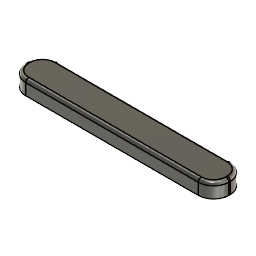
keycapX5 (Autodesk Fusion 360 design; units mm, degrees)
Autodesk Fusion 360 part; units mm, degrees
sketch "Sketch1" plane through (0, 0, 0) normal (0, 0, 1) x (1, 0, 0)
  line L0 (-0.6, 1) -> (-0.6, 2.15)
  line L1 (-0.6, 2.15) -> (0.6, 2.15)
  line L2 (0.6, 2.15) -> (0.6, 1)
  line L3 (0.9, 0.7) -> (2.15, 0.7)
  line L4 (2.15, 0.7) -> (2.15, -0.7)
  line L5 (2.15, -0.7) -> (0.9, -0.7)
  line L6 (0.6, -1) -> (0.6, -2.15)
  line L7 (0.6, -2.15) -> (-0.6, -2.15)
  line L8 (-0.6, -2.15) -> (-0.6, -1)
  line L9 (-0.9, -0.7) -> (-2.15, -0.7)
  line L10 (-2.15, -0.7) -> (-2.15, 0.7)
  line L11 (-2.15, 0.7) -> (-0.9, 0.7)
  arc A0 (-0.9, 0.7) -> (-0.6, 1) centre (-0.9, 1) ccw
  arc A1 (0.6, 1) -> (0.9, 0.7) centre (0.9, 1) ccw
  arc A2 (-0.6, -1) -> (-0.9, -0.7) centre (-0.9, -1) ccw
  arc A3 (0.9, -0.7) -> (0.6, -1) centre (0.9, -1) ccw
  circle A4 centre (0, 0) radius 3
  line L12 (28.9, 0.7) -> (30.15, 0.7)
  line L13 (27.4, 2.15) -> (28.6, 2.15)
  line L14 (28.6, -2.15) -> (27.4, -2.15)
  line L15 (30.15, 0.7) -> (30.15, -0.7)
  line L16 (25.85, -0.7) -> (25.85, 0.7)
  arc A5 (28.9, -0.7) -> (28.6, -1) centre (28.9, -1) ccw
  arc A6 (27.1, 0.7) -> (27.4, 1) centre (27.1, 1) ccw
  line L17 (28.6, 2.15) -> (28.6, 1)
  line L18 (27.4, -2.15) -> (27.4, -1)
  line L19 (30.15, -0.7) -> (28.9, -0.7)
  arc A7 (27.4, -1) -> (27.1, -0.7) centre (27.1, -1) ccw
  arc A8 (28.6, 1) -> (28.9, 0.7) centre (28.9, 1) ccw
  line L20 (27.4, 1) -> (27.4, 2.15)
  line L21 (27.1, -0.7) -> (25.85, -0.7)
  circle A9 centre (28, 0) radius 3
  line L22 (28.6, -1) -> (28.6, -2.15)
  line L23 (25.85, 0.7) -> (27.1, 0.7)
  circle A10 centre (56, 0) radius 3
  line L24 (58.15, -0.7) -> (56.9, -0.7)
  line L25 (55.4, 2.15) -> (56.6, 2.15)
  arc A11 (56.9, -0.7) -> (56.6, -1) centre (56.9, -1) ccw
  arc A12 (55.1, 0.7) -> (55.4, 1) centre (55.1, 1) ccw
  arc A13 (55.4, -1) -> (55.1, -0.7) centre (55.1, -1) ccw
  line L26 (53.85, 0.7) -> (55.1, 0.7)
  arc A14 (56.6, 1) -> (56.9, 0.7) centre (56.9, 1) ccw
  line L27 (56.9, 0.7) -> (58.15, 0.7)
  line L28 (55.4, -2.15) -> (55.4, -1)
  line L29 (56.6, 2.15) -> (56.6, 1)
  line L30 (55.1, -0.7) -> (53.85, -0.7)
  line L31 (55.4, 1) -> (55.4, 2.15)
  line L32 (58.15, 0.7) -> (58.15, -0.7)
  line L33 (53.85, -0.7) -> (53.85, 0.7)
  line L34 (56.6, -1) -> (56.6, -2.15)
  line L35 (56.6, -2.15) -> (55.4, -2.15)
  line L36 (86.15, -0.7) -> (84.9, -0.7)
  line L37 (86.15, 0.7) -> (86.15, -0.7)
  line L38 (81.85, -0.7) -> (81.85, 0.7)
  line L39 (83.4, -2.15) -> (83.4, -1)
  arc A15 (83.1, 0.7) -> (83.4, 1) centre (83.1, 1) ccw
  circle A16 centre (84, 0) radius 3
  line L40 (84.6, -1) -> (84.6, -2.15)
  line L41 (84.6, -2.15) -> (83.4, -2.15)
  line L42 (83.4, 2.15) -> (84.6, 2.15)
  line L43 (81.85, 0.7) -> (83.1, 0.7)
  arc A17 (84.6, 1) -> (84.9, 0.7) centre (84.9, 1) ccw
  line L44 (83.1, -0.7) -> (81.85, -0.7)
  arc A18 (84.9, -0.7) -> (84.6, -1) centre (84.9, -1) ccw
  arc A19 (83.4, -1) -> (83.1, -0.7) centre (83.1, -1) ccw
  line L45 (83.4, 1) -> (83.4, 2.15)
  line L46 (84.9, 0.7) -> (86.15, 0.7)
  line L47 (84.6, 2.15) -> (84.6, 1)
  line L48 (114.15, -0.7) -> (112.9, -0.7)
  line L49 (114.15, 0.7) -> (114.15, -0.7)
  line L50 (109.85, -0.7) -> (109.85, 0.7)
  line L51 (111.4, -2.15) -> (111.4, -1)
  arc A20 (111.1, 0.7) -> (111.4, 1) centre (111.1, 1) ccw
  circle A21 centre (112, 0) radius 3
  line L52 (112.6, -1) -> (112.6, -2.15)
  line L53 (112.6, -2.15) -> (111.4, -2.15)
  line L54 (111.4, 2.15) -> (112.6, 2.15)
  line L55 (109.85, 0.7) -> (111.1, 0.7)
  arc A22 (112.6, 1) -> (112.9, 0.7) centre (112.9, 1) ccw
  line L56 (111.1, -0.7) -> (109.85, -0.7)
  arc A23 (112.9, -0.7) -> (112.6, -1) centre (112.9, -1) ccw
  arc A24 (111.4, -1) -> (111.1, -0.7) centre (111.1, -1) ccw
  line L57 (111.4, 1) -> (111.4, 2.15)
  line L58 (112.9, 0.7) -> (114.15, 0.7)
  line L59 (112.6, 2.15) -> (112.6, 1)
  point P0 (0.6, 0.7)
  point P1 (28.6, 0.7)
  point P2 (28, 0)
  point P3 (56, 0)
  point P4 (56.6, 0.7)
  point P5 (84, 0)
  point P6 (84.6, 0.7)
  point P7 (112, 0)
  point P8 (112.6, 0.7)
  dimension "d2" = 4.3
  dimension "d3" = 4.3
  dimension "d4" = 2.15
  dimension "d5" = 2.15
  dimension "d6" = 1.2
  dimension "d7" = 1.4
  dimension "d8" = 0.7
  dimension "d9" = 0.6
  dimension "d10" = 0.3
  dimension "d11" = 6
  dimension "d36" = 4.3
  dimension "d37" = 4.3
  dimension "d38" = 2.15
  dimension "d39" = 2.15
  dimension "d40" = 1.2
  dimension "d41" = 1.4
  dimension "d42" = 0.7
  dimension "d43" = 0.6
  dimension "d44" = 0.3
  dimension "d45" = 6
  dimension "d46" = 28
  dimension "d47" = 4.3
  dimension "d48" = 4.3
  dimension "d49" = 2.15
  dimension "d50" = 2.15
  dimension "d51" = 1.2
  dimension "d52" = 1.4
  dimension "d53" = 0.7
  dimension "d54" = 0.6
  dimension "d55" = 0.3
  dimension "d56" = 6
  dimension "d57" = 28
  dimension "d58" = 4.3
  dimension "d59" = 4.3
  dimension "d60" = 2.15
  dimension "d61" = 2.15
  dimension "d62" = 1.2
  dimension "d63" = 1.4
  dimension "d64" = 0.7
  dimension "d65" = 0.6
  dimension "d66" = 0.3
  dimension "d67" = 6
  dimension "d68" = 4.3
  dimension "d69" = 4.3
  dimension "d70" = 2.15
  dimension "d71" = 2.15
  dimension "d72" = 1.2
  dimension "d73" = 1.4
  dimension "d74" = 0.7
  dimension "d75" = 0.6
  dimension "d76" = 0.3
  dimension "d77" = 6
  dimension "d78" = 28
  dimension "d79" = 28
  constraint vertical L0
  constraint perpendicular L0 L1
  constraint perpendicular L1 L2
  constraint perpendicular L2 L3
  constraint perpendicular L3 L4
  constraint perpendicular L4 L5
  constraint perpendicular L3 L6
  constraint perpendicular L6 L7
  constraint perpendicular L7 L8
  constraint perpendicular L8 L9
  constraint perpendicular L7 L10
  constraint perpendicular L0 L11
  constraint tangent L0 A0
  constraint tangent L11 A0
  constraint coincident P0 L2
  constraint coincident P0 L3
  constraint tangent L2 A1
  constraint tangent L3 A1
  constraint equal A0 A1
  constraint tangent L8 A2
  constraint tangent L9 A2
  constraint equal A0 A2
  constraint tangent L5 A3
  constraint tangent L6 A3
  constraint equal A0 A3
  constraint horizontal P0 L11.end
  constraint horizontal L9.start L5.end
  constraint vertical L0.start L8.end
  constraint vertical P0 L6.start
  constraint coincident A4.centre origin
  constraint vertical L20
  constraint perpendicular L13 L20
  constraint perpendicular L13 L17
  constraint perpendicular L12 L17
  constraint perpendicular L12 L15
  constraint perpendicular L15 L19
  constraint perpendicular L12 L22
  constraint perpendicular L14 L22
  constraint perpendicular L14 L18
  constraint perpendicular L18 L21
  constraint perpendicular L14 L16
  constraint perpendicular L20 L23
  constraint tangent A6 L20
  constraint tangent A6 L23
  constraint coincident P1 L17
  constraint coincident P1 L12
  constraint tangent L17 A8
  constraint tangent L12 A8
  constraint equal A6 A8
  constraint tangent L18 A7
  constraint tangent A7 L21
  constraint equal A6 A7
  constraint tangent A5 L19
  constraint tangent A5 L22
  constraint equal A5 A6
  constraint horizontal P1 A6.start
  constraint horizontal A7.end A5.start
  constraint vertical A6.end L18.end
  constraint vertical P1 A5.end
  constraint coincident P2 A9.centre
  constraint horizontal A4.centre P2
  constraint vertical L31
  constraint perpendicular L25 L31
  constraint perpendicular L25 L29
  constraint perpendicular L27 L29
  constraint perpendicular L27 L32
  constraint perpendicular L24 L32
  constraint perpendicular L27 L34
  constraint perpendicular L34 L35
  constraint perpendicular L28 L35
  constraint perpendicular L28 L30
  constraint perpendicular L33 L35
  constraint perpendicular L26 L31
  constraint tangent A12 L31
  constraint tangent A12 L26
  constraint coincident P4 L29
  constraint coincident P4 L27
  constraint tangent A14 L29
  constraint tangent A14 L27
  constraint equal A12 A14
  constraint tangent A13 L28
  constraint tangent A13 L30
  constraint equal A12 A13
  constraint tangent L24 A11
  constraint tangent A11 L34
  constraint equal A11 A12
  constraint horizontal A12.start P4
  constraint horizontal L24.end A13.end
  constraint vertical A13.start A12.end
  constraint vertical A11.end P4
  constraint coincident P3 A10.centre
  constraint horizontal P2 P3
  constraint vertical L45
  constraint perpendicular L42 L45
  constraint perpendicular L42 L47
  constraint perpendicular L46 L47
  constraint perpendicular L37 L46
  constraint perpendicular L36 L37
  constraint perpendicular L40 L46
  constraint perpendicular L40 L41
  constraint perpendicular L39 L41
  constraint perpendicular L39 L44
  constraint perpendicular L38 L41
  constraint perpendicular L43 L45
  constraint tangent A15 L45
  constraint tangent A15 L43
  constraint coincident P6 L47
  constraint coincident P6 L46
  constraint tangent A17 L47
  constraint tangent A17 L46
  constraint equal A15 A17
  constraint tangent L39 A19
  constraint tangent L44 A19
  constraint equal A15 A19
  constraint tangent L36 A18
  constraint tangent L40 A18
  constraint equal A15 A18
  constraint horizontal P6 A15.start
  constraint horizontal L44.start L36.end
  constraint vertical A15.end L39.end
  constraint vertical P6 L40.start
  constraint coincident P5 A16.centre
  constraint vertical L57
  constraint perpendicular L54 L57
  constraint perpendicular L54 L59
  constraint perpendicular L58 L59
  constraint perpendicular L49 L58
  constraint perpendicular L48 L49
  constraint perpendicular L52 L58
  constraint perpendicular L52 L53
  constraint perpendicular L51 L53
  constraint perpendicular L51 L56
  constraint perpendicular L50 L53
  constraint perpendicular L55 L57
  constraint tangent A20 L57
  constraint tangent A20 L55
  constraint coincident P8 L59
  constraint coincident P8 L58
  constraint tangent A22 L59
  constraint tangent A22 L58
  constraint equal A20 A22
  constraint tangent L51 A24
  constraint tangent L56 A24
  constraint equal A20 A24
  constraint tangent L48 A23
  constraint tangent L52 A23
  constraint equal A20 A23
  constraint horizontal P8 A20.start
  constraint horizontal L56.start L48.end
  constraint vertical A20.end L51.end
  constraint vertical P8 L52.start
  constraint coincident P7 A21.centre
  constraint horizontal P5 P7
  constraint horizontal P3 P5
  measures "d2" distance of L4 L10
  measures "d3" distance of L1 L7
  measures "d4" distance of A4.centre L4
  measures "d5" distance of A4.centre L7
  measures "d6" distance of L0.end L1.end
  measures "d7" distance of L3.end L4.end
  measures "d8" vertical distance of A4.centre P0
  measures "d9" horizontal distance of A4.centre P0
  measures "d10" radius of A0
  measures "d11" diameter of A4
  measures "d36" distance of L15 L16
  measures "d37" distance of L13 L14
  measures "d38" distance of P2 L15
  measures "d39" distance of P2 L14
  measures "d40" distance of L13.start L13.end
  measures "d41" distance of L12.end L15.end
  measures "d42" vertical distance of P1 P2
  measures "d43" horizontal distance of P1 P2
  measures "d44" radius of A6
  measures "d45" diameter of A9
  measures "d46" distance of A4.centre P2
  measures "d47" distance of L32 L33
  measures "d48" distance of L25 L35
  measures "d49" distance of P3 L32
  measures "d50" distance of P3 L35
  measures "d51" distance of L25.start L25.end
  measures "d52" distance of L27.end L24.start
  measures "d53" vertical distance of P3 P4
  measures "d54" horizontal distance of P3 P4
  measures "d55" radius of A12
  measures "d56" diameter of A10
  measures "d57" distance of P2 P3
  measures "d58" distance of L37 L38
  measures "d59" distance of L41 L42
  measures "d60" distance of P5 L37
  measures "d61" distance of P5 L41
  measures "d62" distance of L42.start L42.end
  measures "d63" distance of L36.start L37.start
  measures "d64" vertical distance of P5 P6
  measures "d65" horizontal distance of P5 P6
  measures "d66" radius of A15
  measures "d67" diameter of A16
  measures "d68" distance of L49 L50
  measures "d69" distance of L53 L54
  measures "d70" distance of P7 L49
  measures "d71" distance of P7 L53
  measures "d72" distance of L54.start L54.end
  measures "d73" distance of L48.start L49.start
  measures "d74" vertical distance of P7 P8
  measures "d75" horizontal distance of P7 P8
  measures "d76" radius of A20
  measures "d77" diameter of A21
  measures "d78" distance of P3 P5
  measures "d79" distance of P5 P7
extrude "Extrude1" add sketch "Sketch1" along normal blind 7 makes body 1 at (2.9851, -0.2987, 4.6667) makes body 2 at (30.9851, -0.2987, 4.6667) makes body 3 at (58.9851, -0.2987, 4.6667) makes body 4 at (84.9555, 2.8438, 4.6667) makes body 5 at (110.6314, -2.6696, 2.3333)
sketch "Sketch2" plane through (0, 0, 7) normal (0, 0, 1) x (-1, 0, 0)
  line L0 (-2.15, 0.7) -> (-0.9, 0.7)
  arc A0 (-0.9, 0.7) -> (-0.6, 1) centre (-0.9, 1) ccw
  line L1 (-0.6, 1) -> (-0.6, 2.15)
  line L2 (-0.6, 2.15) -> (0.6, 2.15)
  line L3 (0.6, 2.15) -> (0.6, 1)
  arc A1 (0.6, 1) -> (0.9, 0.7) centre (0.9, 1) ccw
  line L4 (0.9, 0.7) -> (2.15, 0.7)
  line L5 (2.15, 0.7) -> (2.15, -0.7)
  line L6 (2.15, -0.7) -> (0.9, -0.7)
  arc A2 (0.9, -0.7) -> (0.6, -1) centre (0.9, -1) ccw
  line L7 (0.6, -1) -> (0.6, -2.15)
  line L8 (0.6, -2.15) -> (-0.6, -2.15)
  line L9 (-0.6, -2.15) -> (-0.6, -1)
  arc A3 (-0.6, -1) -> (-0.9, -0.7) centre (-0.9, -1) ccw
  line L10 (-0.9, -0.7) -> (-2.15, -0.7)
  line L11 (-2.15, -0.7) -> (-2.15, 0.7)
  circle A4 centre (0, 0) radius 3
  line L12 (10.5, 10.5) -> (-122.5, 10.5)
  line L13 (-122.5, 10.5) -> (-122.5, -10.5)
  line L14 (-122.5, -10.5) -> (10.5, -10.5)
  line L15 (10.5, -10.5) -> (10.5, 10.5)
  dimension "d14" = 133
  dimension "d15" = 21
  dimension "d16" = 10.5
  dimension "d17" = 10.5
  constraint horizontal L12
  constraint vertical L13
  constraint horizontal L14
  constraint vertical L15
  measures "d14" distance of L12.start L12.end
  measures "d15" distance of L12.start L14.end
  measures "d16" horizontal distance of A4.centre L12.start
  measures "d17" vertical distance of A4.centre L12.start
extrude "Extrude2" add sketch "Sketch2" along normal blind 2 contours L0 A0 L1 L2 L3 A1 L4 L5 L6 A2 L7 L8 L9 A3 L10 L11 | A4 | L12 L13 L14 L15 bodies 1 2
sketch "Sketch3" plane through (0, 0, 7) normal (0, 0, -1) x (1, 0, 0)
  line L0 (-10.5, 10.5) -> (-10.5, -10.5)
  line L1 (-10.5, -10.5) -> (122.5, -10.5)
  line L2 (122.5, -10.5) -> (122.5, 10.5)
  line L3 (122.5, 10.5) -> (-10.5, 10.5)
  circle A0 centre (0, 0) radius 3
  line L4 (122.5, -10.5) -> (-10.5, -10.5)
  line L5 (-10.5, -10.5) -> (-10.5, 10.5)
  line L6 (-10.5, 10.5) -> (122.5, 10.5)
  line L7 (122.5, 10.5) -> (122.5, -10.5)
  line L8 (-8.9, 8.9) -> (120.9, 8.9)
  line L9 (120.9, 8.9) -> (120.9, -8.9)
  line L10 (120.9, -8.9) -> (-8.9, -8.9)
  line L11 (-8.9, -8.9) -> (-8.9, 8.9)
  circle A1 centre (28, 0) radius 3
  dimension "d20" = 1.6
  dimension "d21" = 1.6
  dimension "d22" = 1.6
  dimension "d23" = 1.6
  constraint horizontal L4
  constraint vertical L5
  constraint horizontal L6
  constraint vertical L7
  constraint coincident L0.start L3.end
  constraint coincident L1.end L2.start
  constraint horizontal L8
  constraint vertical L9
  constraint horizontal L10
  constraint vertical L11
  measures "d20" vertical distance of L1.end L9.end
  measures "d21" horizontal distance of L1.end L9.end
  measures "d22" horizontal distance of L0.end L10.end
  measures "d23" vertical distance of L0.start L8.start
extrude "Extrude3" add sketch "Sketch3" along normal blind 7.5 contours L0 L1 L2 L3 L4 L5 L6 L7 bodies 1
fillet "Fillet1" radius 3 1 faces at (90.9333, 0, 7) on bodies 1
fillet "Fillet1" radius 8.4 4 edges at (-8.9, -8.9, 3.25) (-8.9, 8.9, 3.25) (120.9, 8.9, 3.25) (120.9, -8.9, 3.25) on bodies 1
fillet "Fillet1" radius 10 4 edges at (-10.5, -10.5, 4.25) (-10.5, 10.5, 4.25) (122.5, -10.5, 4.25) (122.5, 10.5, 4.25) on bodies 1
fillet "Fillet1" radius 2 1 faces at (78.1667, -3.5, 9) on bodies 1
extrude "Extrude4" add 2 faces at (-0.2345, 0.2578, 7) (27.7655, -0.2578, 7) along direction (0, 0, -1) blind 3.3 on bodies 1 bodies 1
equation "d8 = ( 1.4 / 2 ) * 1 mm"
equation "d9 = ( 1.2 / 2 ) * 1 mm"
equation "d14 = ( ( 28 * 4 ) * 1 mm ) + 21 mm"
equation "d16 = ( 21 / 2 ) * 1 mm"
equation "d17 = ( 21 / 2 ) * 1 mm"
equation "d34 = 7 mm - 3.7 mm"
equation "d42 = ( 1.4 / 2 ) * 1 mm"
equation "d43 = ( 1.2 / 2 ) * 1 mm"
equation "d53 = ( 1.4 / 2 ) * 1 mm"
equation "d54 = ( 1.2 / 2 ) * 1 mm"
equation "d64 = ( 1.4 / 2 ) * 1 mm"
equation "d65 = ( 1.2 / 2 ) * 1 mm"
equation "d74 = ( 1.4 / 2 ) * 1 mm"
equation "d75 = ( 1.2 / 2 ) * 1 mm"
